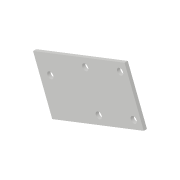
# Autodesk Inventor part: VWheelArmThick
Saved by Autodesk Inventor 2018 (Build 220112000, 112)
## iProperties
Created: 2018-12-14
Part Number: VWheelArmThick
Material: Generic
Document SubType Name: Modeling
Designer: ball
Density: 1 g/cm^3
Appearance: Default
Author: ball
Autodesk Inventor part; units mm, degrees
ref_plane "YZ Plane" through (0, 0, 0) normal (1, 0, 0) x (0, 1, 0)
ref_plane "XZ Plane" through (0, 0, 0) normal (0, 1, 0) x (-1, 0, 0)
ref_plane "XY Plane" through (0, 0, 0) normal (0, 0, 1) x (1, 0, 0)
sketch "Sketch1" plane through (0, 0, 0) normal (0, 0, 1) x (1, 0, 0)
  circle A0 centre (50.1681, 27.2834) radius 1.778 construction
  circle A1 centre (25.0574, 17.5233) radius 1.778 construction
  circle A2 centre (34.8176, -7.5874) radius 1.778 construction
  circle A3 centre (59.9282, 2.1728) radius 1.778 construction
  circle A4 centre (0, 0) radius 3.5 construction
  circle A5 centre (44.7061, 31.1467) radius 1.778 construction
  circle A6 centre (58.509, -4.3651) radius 1.778 construction
  circle A7 centre (26.4767, 24.0612) radius 1.778 construction
  circle A8 centre (40.2796, -11.4506) radius 1.778 construction
  line L0 (44.7061, 31.1467) -> (26.4767, 24.0612) construction
  line L1 (58.509, -4.3651) -> (40.2796, -11.4506) construction
  line L2 (168.5413, -268.1733) -> (30.5122, 86.945) construction
  circle A9 centre (-14.8554, 15.0432) radius 1.778 construction
  circle A10 centre (1.8062, -27.8234) radius 1.778 construction
  line L3 (67.1502, -1.0064) -> (1.3271, -26.5908)
  line L4 (53.3473, 34.5054) -> (-12.4758, 8.921)
  line L5 (-12.4758, 8.921) -> (1.3271, -26.5908)
  circle A11 centre (50.1681, 27.2834) radius 2.2479
  circle A12 centre (59.9282, 2.1728) radius 2.2479
  circle A13 centre (34.8176, -7.5874) radius 2.2479
  circle A14 centre (25.0574, 17.5233) radius 2.2479
  circle A15 centre (0, 0) radius 2.2479
  line L6 (53.3473, 34.5054) -> (67.1502, -1.0064)
  point P0 (51.2166, 33.6772)
  dimension "d0" = 4.4958
  dimension "d1" = 4.4958
  dimension "d2" = 4.4958
  dimension "d3" = 4.4958
  dimension "d4" = 4.4958
  constraints: 16 centre point, 14 end point, 5 coincident, 4 point on line, 28 other
  measures "d0" diameter of A11
  measures "d1" diameter of A12
  measures "d2" diameter of A13
  measures "d3" diameter of A14
  measures "d4" diameter of A15
extrude "Extrusion1" add sketch "Sketch1" along normal blind 2.286
body "Solid1"
